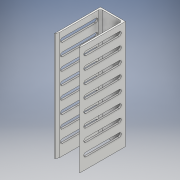
# Autodesk Inventor part: LiFeGuard
Saved by Autodesk Inventor 2018 (Build 220112000, 112)
## iProperties
Created: 2018-08-27
Part Number: LiFeGuard
Material: ABS プラスチック
Document SubType Name: Modeling
Designer: shun2
Density: 1.06 g/cm^3
Appearance: 滑らか - 白
Author: shun2
Autodesk Inventor part; units mm, degrees
ref_plane "YZ Plane" through (0, 0, 0) normal (1, 0, 0) x (0, 1, 0)
ref_plane "XZ Plane" through (0, 0, 0) normal (0, 1, 0) x (-1, 0, 0)
ref_plane "XY Plane" through (0, 0, 0) normal (0, 0, 1) x (1, 0, 0)
sketch "スケッチ1" plane through (0, 0, 0) normal (0, 0, 1) x (1, 0, 0)
  line L0 (30, 0) -> (30, 55)
  line L1 (30, 55) -> (0, 55)
  line L2 (0, 55) -> (0, 2)
  line L3 (2, 53) -> (2, 2)
  line L4 (2, 2) -> (28, 2)
  line L5 (28, 53) -> (28, 2)
  line L6 (2, 53) -> (28, 53)
  line L7 (0, 2) -> (0, 0)
  line L8 (2, 2) -> (0, 0)
  line L9 (28, 2) -> (30, 0)
  constraints: 20 end point, 3 perpendicular, 1 parallel, 1 vertical
extrude "押し出し1" add sketch "スケッチ1" along normal blind 130 contours L9 L5 L6 L3 L8 L7 L2 L1 L0
sketch "スケッチ2" plane through (30, 0, 0) normal (1, 0, 0) x (0, 0, -1)
  line L0 (-130, 53) -> (-130, 2) projected
  line L1 (-120.6035, 50) -> (-120.6035, 50)
  line L2 (-118.1035, 47.5) -> (-118.1035, 7.5)
  line L3 (-120.6035, 5) -> (-120.6035, 5)
  line L4 (-123.1035, 7.5) -> (-123.1035, 47.5)
  line L5 (-105.6035, 50) -> (-103.1035, 50)
  line L6 (-103.1035, 47.5) -> (-103.1035, 7.5)
  line L7 (-105.6035, 5) -> (-105.6035, 5)
  line L8 (-108.1035, 7.5) -> (-108.1035, 47.5)
  line L9 (-90.6035, 50) -> (-90.6035, 50)
  line L10 (-88.1035, 47.5) -> (-88.1035, 7.5)
  line L11 (-90.6035, 5) -> (-90.6035, 5)
  line L12 (-93.1035, 7.5) -> (-93.1035, 47.5)
  line L13 (-75.6035, 50) -> (-73.1035, 50)
  line L14 (-73.1035, 47.5) -> (-73.1035, 7.5)
  line L15 (-75.6035, 5) -> (-75.6035, 5)
  line L16 (-78.1035, 7.5) -> (-78.1035, 47.5)
  line L17 (-60.6035, 50) -> (-58.1035, 50)
  line L18 (-58.1035, 47.5) -> (-58.1035, 7.5)
  line L19 (-60.6035, 5) -> (-60.6035, 5)
  line L20 (-63.1035, 7.5) -> (-63.1035, 47.5)
  line L21 (-45.6035, 50) -> (-43.1035, 50)
  line L22 (-43.1035, 47.5) -> (-43.1035, 7.5)
  line L23 (-45.6035, 5) -> (-48.1035, 5)
  line L24 (-48.1035, 7.5) -> (-48.1035, 47.5)
  line L25 (-30.6035, 50) -> (-30.6035, 50)
  line L26 (-28.1035, 47.5) -> (-28.1035, 7.5)
  line L27 (-30.6035, 5) -> (-30.6035, 5)
  line L28 (-33.1035, 7.5) -> (-33.1035, 47.5)
  line L29 (-15.6035, 50) -> (-15.6035, 50)
  line L30 (-13.1035, 47.5) -> (-13.1035, 7.5)
  line L31 (-13.1035, 5) -> (-15.6035, 5)
  line L32 (-18.1035, 7.5) -> (-18.1035, 47.5)
  line L33 (-123.1035, 50) -> (-118.1035, 50)
  line L34 (-108.1035, 50) -> (-105.6035, 50)
  line L35 (-93.1035, 50) -> (-88.1035, 50)
  line L36 (-78.1035, 50) -> (-75.6035, 50)
  line L37 (-63.1035, 50) -> (-60.6035, 50)
  line L38 (-48.1035, 50) -> (-45.6035, 50)
  line L39 (-33.1035, 50) -> (-28.1035, 50)
  line L40 (-18.1035, 50) -> (-13.1035, 50)
  line L41 (-18.1035, 5) -> (-15.6035, 5)
  line L42 (-33.1035, 5) -> (-28.1035, 5)
  line L43 (-45.6035, 5) -> (-43.1035, 5)
  line L44 (-63.1035, 5) -> (-58.1035, 5)
  line L45 (-78.1035, 5) -> (-73.1035, 5)
  line L46 (-93.1035, 5) -> (-88.1035, 5)
  line L47 (-123.1035, 5) -> (-118.1035, 5)
  line L48 (-108.1035, 5) -> (-103.1035, 5)
  arc A0 (-120.6035, 50) -> (-123.1035, 47.5) centre (-120.6035, 47.5) ccw
  arc A1 (-118.1035, 47.5) -> (-120.6035, 50) centre (-120.6035, 47.5) ccw
  arc A2 (-105.6035, 50) -> (-108.1035, 47.5) centre (-105.6035, 47.5) ccw
  arc A3 (-103.1035, 47.5) -> (-105.6035, 50) centre (-105.6035, 47.5) ccw
  arc A4 (-90.6035, 50) -> (-93.1035, 47.5) centre (-90.6035, 47.5) ccw
  arc A5 (-88.1035, 47.5) -> (-90.6035, 50) centre (-90.6035, 47.5) ccw
  arc A6 (-75.6035, 50) -> (-78.1035, 47.5) centre (-75.6035, 47.5) ccw
  arc A7 (-73.1035, 47.5) -> (-75.6035, 50) centre (-75.6035, 47.5) ccw
  arc A8 (-60.6035, 50) -> (-63.1035, 47.5) centre (-60.6035, 47.5) ccw
  arc A9 (-58.1035, 47.5) -> (-60.6035, 50) centre (-60.6035, 47.5) ccw
  arc A10 (-45.6035, 50) -> (-48.1035, 47.5) centre (-45.6035, 47.5) ccw
  arc A11 (-43.1035, 47.5) -> (-45.6035, 50) centre (-45.6035, 47.5) ccw
  arc A12 (-30.6035, 50) -> (-33.1035, 47.5) centre (-30.6035, 47.5) ccw
  arc A13 (-28.1035, 47.5) -> (-30.6035, 50) centre (-30.6035, 47.5) ccw
  arc A14 (-15.6035, 50) -> (-18.1035, 47.5) centre (-15.6035, 47.5) ccw
  arc A15 (-13.1035, 47.5) -> (-15.6035, 50) centre (-15.6035, 47.5) ccw
  arc A16 (-18.1035, 7.5) -> (-15.6035, 5) centre (-15.6035, 7.5) ccw
  arc A17 (-15.6035, 5) -> (-13.1035, 7.5) centre (-15.6035, 7.5) ccw
  arc A18 (-30.6035, 5) -> (-28.1035, 7.5) centre (-30.6035, 7.5) ccw
  arc A19 (-33.1035, 7.5) -> (-30.6035, 5) centre (-30.6035, 7.5) ccw
  arc A20 (-45.6035, 5) -> (-43.1035, 7.5) centre (-45.6035, 7.5) ccw
  arc A21 (-48.1035, 7.5) -> (-45.6035, 5) centre (-45.6035, 7.5) ccw
  arc A22 (-60.6035, 5) -> (-58.1035, 7.5) centre (-60.6035, 7.5) ccw
  arc A23 (-63.1035, 7.5) -> (-60.6035, 5) centre (-60.6035, 7.5) ccw
  arc A24 (-75.6035, 5) -> (-73.1035, 7.5) centre (-75.6035, 7.5) ccw
  arc A25 (-78.1035, 7.5) -> (-75.6035, 5) centre (-75.6035, 7.5) ccw
  arc A26 (-90.6035, 5) -> (-88.1035, 7.5) centre (-90.6035, 7.5) ccw
  arc A27 (-93.1035, 7.5) -> (-90.6035, 5) centre (-90.6035, 7.5) ccw
  arc A28 (-108.1035, 7.5) -> (-105.6035, 5) centre (-105.6035, 7.5) ccw
  arc A29 (-105.6035, 5) -> (-103.1035, 7.5) centre (-105.6035, 7.5) ccw
  arc A30 (-120.6035, 5) -> (-118.1035, 7.5) centre (-120.6035, 7.5) ccw
  arc A31 (-123.1035, 7.5) -> (-120.6035, 5) centre (-120.6035, 7.5) ccw
  line L49 (-108.1035, 47.5) -> (-108.1035, 7.5)
  line L50 (-103.1035, 7.5) -> (-103.1035, 47.5)
  line L51 (-78.1035, 47.5) -> (-78.1035, 7.5)
  line L52 (-73.1035, 7.5) -> (-73.1035, 47.5)
  line L53 (-48.1035, 47.5) -> (-48.1035, 7.5)
  line L54 (-43.1035, 7.5) -> (-43.1035, 47.5)
  line L55 (-33.1035, 47.5) -> (-33.1035, 7.5)
  line L56 (-28.1035, 7.5) -> (-28.1035, 47.5)
  circle A32 centre (-105.6035, 47.5) radius 2.5
  circle A33 centre (-90.6035, 47.5) radius 2.5
  circle A34 centre (-75.6035, 47.5) radius 2.5
  circle A35 centre (-60.6035, 47.5) radius 2.5
  circle A36 centre (-45.6035, 47.5) radius 2.5
  circle A37 centre (-30.6035, 47.5) radius 2.5
  circle A38 centre (-15.6035, 47.5) radius 2.5
  circle A39 centre (-15.6035, 7.5) radius 2.5
  circle A40 centre (-30.6035, 7.5) radius 2.5
  circle A41 centre (-45.6035, 7.5) radius 2.5
  circle A42 centre (-60.6035, 7.5) radius 2.5
  circle A43 centre (-75.6035, 7.5) radius 2.5
  circle A44 centre (-90.6035, 7.5) radius 2.5
  circle A45 centre (-105.6035, 7.5) radius 2.5
  circle A46 centre (-120.6035, 7.5) radius 2.5
  line L57 (-108.1035, 47.5) -> (-108.1035, 7.5)
  line L58 (-103.1035, 7.5) -> (-103.1035, 47.5)
  line L59 (-93.1035, 47.5) -> (-93.1035, 7.5)
  line L60 (-88.1035, 7.5) -> (-88.1035, 47.5)
  line L61 (-78.1035, 47.5) -> (-78.1035, 7.5)
  line L62 (-73.1035, 7.5) -> (-73.1035, 47.5)
  line L63 (-63.1035, 47.5) -> (-63.1035, 7.5)
  line L64 (-58.1035, 7.5) -> (-58.1035, 47.5)
  line L65 (-48.1035, 47.5) -> (-48.1035, 7.5)
  line L66 (-43.1035, 7.5) -> (-43.1035, 47.5)
  line L67 (-33.1035, 47.5) -> (-33.1035, 7.5)
  line L68 (-28.1035, 7.5) -> (-28.1035, 47.5)
  line L69 (-18.1035, 47.5) -> (-18.1035, 7.5)
  line L70 (-13.1035, 7.5) -> (-13.1035, 47.5)
  line L71 (-108.1035, 47.5) -> (-103.1035, 47.5)
  line L72 (-103.1035, 47.5) -> (-103.1035, 7.5)
  line L73 (-103.1035, 7.5) -> (-108.1035, 7.5)
  line L74 (-108.1035, 7.5) -> (-108.1035, 47.5)
  line L75 (-93.1035, 7.5) -> (-88.1035, 7.5)
  line L76 (-88.1035, 7.5) -> (-88.1035, 47.5)
  line L77 (-88.1035, 47.5) -> (-93.1035, 47.5)
  line L78 (-93.1035, 47.5) -> (-93.1035, 7.5)
  line L79 (-78.1035, 47.5) -> (-73.1035, 47.5)
  line L80 (-73.1035, 47.5) -> (-73.1035, 7.5)
  line L81 (-73.1035, 7.5) -> (-78.1035, 7.5)
  line L82 (-78.1035, 7.5) -> (-78.1035, 47.5)
  line L83 (-63.1035, 7.5) -> (-58.1035, 7.5)
  line L84 (-58.1035, 7.5) -> (-58.1035, 47.5)
  line L85 (-58.1035, 47.5) -> (-63.1035, 47.5)
  line L86 (-63.1035, 47.5) -> (-63.1035, 7.5)
  line L87 (-48.1035, 47.5) -> (-43.1035, 47.5)
  line L88 (-43.1035, 47.5) -> (-43.1035, 7.5)
  line L89 (-43.1035, 7.5) -> (-48.1035, 7.5)
  line L90 (-48.1035, 7.5) -> (-48.1035, 47.5)
  line L91 (-33.1035, 7.5) -> (-28.1035, 7.5)
  line L92 (-28.1035, 7.5) -> (-28.1035, 47.5)
  line L93 (-28.1035, 47.5) -> (-33.1035, 47.5)
  line L94 (-33.1035, 47.5) -> (-33.1035, 7.5)
  line L95 (-18.1035, 47.5) -> (-13.1035, 47.5)
  line L96 (-13.1035, 47.5) -> (-13.1035, 7.5)
  line L97 (-13.1035, 7.5) -> (-18.1035, 7.5)
  line L98 (-18.1035, 7.5) -> (-18.1035, 47.5)
  point P0 (0, 0)
  point P1 (-44, 28.2547)
  dimension "d8" = 5
  dimension "d9" = 5
  dimension "d10" = 5
  dimension "d11" = 5
  dimension "d12" = 5
  dimension "d13" = 5
  dimension "d14" = 5
  dimension "d15" = 10
  dimension "d16" = 10
  dimension "d17" = 10
  dimension "d18" = 10
  dimension "d19" = 10
  dimension "d20" = 10
  dimension "d21" = 5
  dimension "d22" = 10
  dimension "d31" = 2.5
  constraints: 196 end point, 64 point on circle, 64 point on line, 64 tangent, 40 parallel, 32 centre point, 31 equal radius, 23 horizontal, 15 coincident, 15 horizontal alignment, 15 perpendicular, 10 collinear, 4 vertical, 30 other
  measures "d8" distance of L47.start L47.end
  measures "d9" distance of L48.end L48.start
  measures "d10" distance of L46.end L46.start
  measures "d11" distance of L45.end L45.start
  measures "d12" distance of L44.end L44.start
  measures "d13" distance of L43.end L23.end
  measures "d14" distance of L42.end L42.start
  measures "d15" distance between parallel lines of L8 L2
  measures "d16" distance between parallel lines of L12 L6
  measures "d17" distance between parallel lines of L16 L10
  measures "d18" distance between parallel lines of L20 L14
  measures "d19" distance between parallel lines of L24 L18
  measures "d20" distance between parallel lines of L28 L22
  measures "d21" distance of L31.start L41.start
  measures "d22" distance between parallel lines of L32 L26
  measures "d31" radius of A0
chamfer "面取り1" distance 2 angle 45 2 edges at (2, 53, 65) (28, 2, 65)
chamfer "面取り2" distance 2 angle 45 2 edges at (28, 53, 65) (2, 2, 65)
sketch "スケッチ3" plane through (30, 0, 0) normal (1, 0, 0) x (0, 0, -1)
  line L0 (-130, 53) -> (-130, 2)
  line L1 (-120.6035, 50) -> (-120.6035, 50)
  line L2 (-118.1035, 47.5) -> (-118.1035, 7.5)
  line L3 (-120.6035, 5) -> (-120.6035, 5)
  line L4 (-123.1035, 7.5) -> (-123.1035, 47.5)
  line L5 (-105.6035, 50) -> (-103.1035, 50)
  line L6 (-103.1035, 47.5) -> (-103.1035, 7.5)
  line L7 (-105.6035, 5) -> (-105.6035, 5)
  line L8 (-108.1035, 7.5) -> (-108.1035, 47.5)
  line L9 (-90.6035, 50) -> (-90.6035, 50)
  line L10 (-88.1035, 47.5) -> (-88.1035, 7.5)
  line L11 (-90.6035, 5) -> (-90.6035, 5)
  line L12 (-93.1035, 7.5) -> (-93.1035, 47.5)
  line L13 (-75.6035, 50) -> (-73.1035, 50)
  line L14 (-73.1035, 47.5) -> (-73.1035, 7.5)
  line L15 (-75.6035, 5) -> (-75.6035, 5)
  line L16 (-78.1035, 7.5) -> (-78.1035, 47.5)
  line L17 (-60.6035, 50) -> (-58.1035, 50)
  line L18 (-58.1035, 47.5) -> (-58.1035, 7.5)
  line L19 (-60.6035, 5) -> (-60.6035, 5)
  line L20 (-63.1035, 7.5) -> (-63.1035, 47.5)
  line L21 (-45.6035, 50) -> (-43.1035, 50)
  line L22 (-43.1035, 47.5) -> (-43.1035, 7.5)
  line L23 (-45.6035, 5) -> (-48.1035, 5)
  line L24 (-48.1035, 7.5) -> (-48.1035, 47.5)
  line L25 (-30.6035, 50) -> (-30.6035, 50)
  line L26 (-28.1035, 47.5) -> (-28.1035, 7.5)
  line L27 (-30.6035, 5) -> (-30.6035, 5)
  line L28 (-33.1035, 7.5) -> (-33.1035, 47.5)
  line L29 (-15.6035, 50) -> (-15.6035, 50)
  line L30 (-13.1035, 47.5) -> (-13.1035, 7.5)
  line L31 (-13.1035, 5) -> (-15.6035, 5)
  line L32 (-18.1035, 7.5) -> (-18.1035, 47.5)
  line L33 (-123.1035, 50) -> (-118.1035, 50)
  line L34 (-108.1035, 50) -> (-105.6035, 50)
  line L35 (-93.1035, 50) -> (-88.1035, 50)
  line L36 (-78.1035, 50) -> (-75.6035, 50)
  line L37 (-63.1035, 50) -> (-60.6035, 50)
  line L38 (-48.1035, 50) -> (-45.6035, 50)
  line L39 (-33.1035, 50) -> (-28.1035, 50)
  line L40 (-18.1035, 50) -> (-13.1035, 50)
  line L41 (-18.1035, 5) -> (-15.6035, 5)
  line L42 (-33.1035, 5) -> (-28.1035, 5)
  line L43 (-45.6035, 5) -> (-43.1035, 5)
  line L44 (-63.1035, 5) -> (-58.1035, 5)
  line L45 (-78.1035, 5) -> (-73.1035, 5)
  line L46 (-93.1035, 5) -> (-88.1035, 5)
  line L47 (-123.1035, 5) -> (-118.1035, 5)
  line L48 (-108.1035, 5) -> (-103.1035, 5)
  arc A0 (-120.6035, 50) -> (-123.1035, 47.5) centre (-120.6035, 47.5) ccw
  arc A1 (-118.1035, 47.5) -> (-120.6035, 50) centre (-120.6035, 47.5) ccw
  arc A2 (-105.6035, 50) -> (-108.1035, 47.5) centre (-105.6035, 47.5) ccw
  arc A3 (-103.1035, 47.5) -> (-105.6035, 50) centre (-105.6035, 47.5) ccw
  arc A4 (-90.6035, 50) -> (-93.1035, 47.5) centre (-90.6035, 47.5) ccw
  arc A5 (-88.1035, 47.5) -> (-90.6035, 50) centre (-90.6035, 47.5) ccw
  arc A6 (-75.6035, 50) -> (-78.1035, 47.5) centre (-75.6035, 47.5) ccw
  arc A7 (-73.1035, 47.5) -> (-75.6035, 50) centre (-75.6035, 47.5) ccw
  arc A8 (-60.6035, 50) -> (-63.1035, 47.5) centre (-60.6035, 47.5) ccw
  arc A9 (-58.1035, 47.5) -> (-60.6035, 50) centre (-60.6035, 47.5) ccw
  arc A10 (-45.6035, 50) -> (-48.1035, 47.5) centre (-45.6035, 47.5) ccw
  arc A11 (-43.1035, 47.5) -> (-45.6035, 50) centre (-45.6035, 47.5) ccw
  arc A12 (-30.6035, 50) -> (-33.1035, 47.5) centre (-30.6035, 47.5) ccw
  arc A13 (-28.1035, 47.5) -> (-30.6035, 50) centre (-30.6035, 47.5) ccw
  arc A14 (-15.6035, 50) -> (-18.1035, 47.5) centre (-15.6035, 47.5) ccw
  arc A15 (-13.1035, 47.5) -> (-15.6035, 50) centre (-15.6035, 47.5) ccw
  arc A16 (-18.1035, 7.5) -> (-15.6035, 5) centre (-15.6035, 7.5) ccw
  arc A17 (-15.6035, 5) -> (-13.1035, 7.5) centre (-15.6035, 7.5) ccw
  arc A18 (-30.6035, 5) -> (-28.1035, 7.5) centre (-30.6035, 7.5) ccw
  arc A19 (-33.1035, 7.5) -> (-30.6035, 5) centre (-30.6035, 7.5) ccw
  arc A20 (-45.6035, 5) -> (-43.1035, 7.5) centre (-45.6035, 7.5) ccw
  arc A21 (-48.1035, 7.5) -> (-45.6035, 5) centre (-45.6035, 7.5) ccw
  arc A22 (-60.6035, 5) -> (-58.1035, 7.5) centre (-60.6035, 7.5) ccw
  arc A23 (-63.1035, 7.5) -> (-60.6035, 5) centre (-60.6035, 7.5) ccw
  arc A24 (-75.6035, 5) -> (-73.1035, 7.5) centre (-75.6035, 7.5) ccw
  arc A25 (-78.1035, 7.5) -> (-75.6035, 5) centre (-75.6035, 7.5) ccw
  arc A26 (-90.6035, 5) -> (-88.1035, 7.5) centre (-90.6035, 7.5) ccw
  arc A27 (-93.1035, 7.5) -> (-90.6035, 5) centre (-90.6035, 7.5) ccw
  arc A28 (-108.1035, 7.5) -> (-105.6035, 5) centre (-105.6035, 7.5) ccw
  arc A29 (-105.6035, 5) -> (-103.1035, 7.5) centre (-105.6035, 7.5) ccw
  arc A30 (-120.6035, 5) -> (-118.1035, 7.5) centre (-120.6035, 7.5) ccw
  arc A31 (-123.1035, 7.5) -> (-120.6035, 5) centre (-120.6035, 7.5) ccw
  line L49 (-108.1035, 47.5) -> (-108.1035, 7.5)
  line L50 (-103.1035, 7.5) -> (-103.1035, 47.5)
  line L51 (-78.1035, 47.5) -> (-78.1035, 7.5)
  line L52 (-73.1035, 7.5) -> (-73.1035, 47.5)
  line L53 (-48.1035, 47.5) -> (-48.1035, 7.5)
  line L54 (-43.1035, 7.5) -> (-43.1035, 47.5)
  line L55 (-33.1035, 47.5) -> (-33.1035, 7.5)
  line L56 (-28.1035, 7.5) -> (-28.1035, 47.5)
  circle A32 centre (-105.6035, 47.5) radius 2.5
  circle A33 centre (-90.6035, 47.5) radius 2.5
  circle A34 centre (-75.6035, 47.5) radius 2.5
  circle A35 centre (-60.6035, 47.5) radius 2.5
  circle A36 centre (-45.6035, 47.5) radius 2.5
  circle A37 centre (-30.6035, 47.5) radius 2.5
  circle A38 centre (-15.6035, 47.5) radius 2.5
  circle A39 centre (-15.6035, 7.5) radius 2.5
  circle A40 centre (-30.6035, 7.5) radius 2.5
  circle A41 centre (-45.6035, 7.5) radius 2.5
  circle A42 centre (-60.6035, 7.5) radius 2.5
  circle A43 centre (-75.6035, 7.5) radius 2.5
  circle A44 centre (-90.6035, 7.5) radius 2.5
  circle A45 centre (-105.6035, 7.5) radius 2.5
  circle A46 centre (-120.6035, 7.5) radius 2.5
  line L57 (-93.1035, 47.5) -> (-88.1035, 47.5)
  line L58 (-88.1035, 47.5) -> (-88.1035, 7.5)
  line L59 (-88.1035, 7.5) -> (-93.1035, 7.5)
  line L60 (-93.1035, 7.5) -> (-93.1035, 47.5)
  circle A47 centre (-90.6035, 47.5) radius 2.5
  circle A48 centre (-90.6035, 7.5) radius 2.5
  circle A49 centre (-30.6035, 7.5) radius 2.5
  line L61 (-33.1035, 47.5) -> (-28.1035, 47.5)
  line L62 (-28.1035, 47.5) -> (-28.1035, 7.5)
  line L63 (-28.1035, 7.5) -> (-33.1035, 7.5)
  line L64 (-33.1035, 7.5) -> (-33.1035, 47.5)
  circle A50 centre (-30.6035, 47.5) radius 2.5
  point P0 (0, 0)
  point P1 (-44, 28.2547)
  dimension "d34" = 5
  dimension "d35" = 5
  dimension "d36" = 5
  dimension "d37" = 5
  dimension "d38" = 5
  dimension "d39" = 5
  dimension "d40" = 5
  dimension "d41" = 10
  dimension "d42" = 10
  dimension "d43" = 10
  dimension "d44" = 10
  dimension "d45" = 10
  dimension "d46" = 10
  dimension "d47" = 5
  dimension "d48" = 10
  dimension "d49" = 2.5
  constraints: 130 end point, 64 point on circle, 64 point on line, 64 tangent, 32 centre point, 31 equal radius, 22 parallel, 19 coincident, 19 horizontal alignment, 18 horizontal, 10 perpendicular, 6 collinear, 38 other
  measures "d34" distance of L47.start L47.end
  measures "d35" distance of L48.end L48.start
  measures "d36" distance of L46.end L46.start
  measures "d37" distance of L45.end L45.start
  measures "d38" distance of L44.end L44.start
  measures "d39" distance of L43.end L23.end
  measures "d40" distance of L42.end L42.start
  measures "d41" distance between parallel lines of L8 L2
  measures "d42" distance between parallel lines of L12 L6
  measures "d43" distance between parallel lines of L16 L10
  measures "d44" distance between parallel lines of L20 L14
  measures "d45" distance between parallel lines of L24 L18
  measures "d46" distance between parallel lines of L28 L22
  measures "d47" distance of L31.start L41.start
  measures "d48" distance between parallel lines of L32 L26
  measures "d49" radius of A0
extrude "押し出し3" cut sketch "スケッチ2" against normal blind 300
extrude "押し出し4" cut sketch "スケッチ3" against normal blind 300 contours L57 A4 A5 | L10 A44 L12 A33 | A33 L57 | L59 A44 | A26 A27 L59 | L61 A12 A13 | L26 A40 L28 A37 | A37 L61 | L63 A40 | A18 A19 L63
